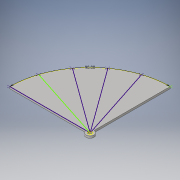
# Autodesk Inventor part: swiweller
Saved by Autodesk Inventor 2016 SP2 (Build 200236200, 236)
## iProperties
Created: 2017-09-03
Part Number: swiweller
Material: Generic
Document SubType Name: Modeling
Designer: Kartikye
Density: 1 g/cm^3
Appearance: Default
Author: Kartikye
Autodesk Inventor part; units mm, degrees
ref_plane "YZ Plane" through (0, 0, 0) normal (1, 0, 0) x (0, 1, 0)
ref_plane "XZ Plane" through (0, 0, 0) normal (0, 1, 0) x (-1, 0, 0)
ref_plane "XY Plane" through (0, 0, 0) normal (0, 0, 1) x (1, 0, 0)
sketch "Sketch5" plane through (0, 0, 0) normal (0, 1, 0) x (-1, 0, 0)
  line L0 (0, 0) -> (127, 0) construction
  circle A0 centre (0, 0) radius 127
  line L1 (0, 0) -> (127, 0)
  line L2 (0, 0) -> (0, -127)
  dimension "d27" = 254
  constraints: 6 end point, 2 horizontal, 1 coincident, 1 vertical, 1 vertical alignment, 2 other
extrude "Extrusion2" add sketch "Sketch5" along normal blind 3.175
sketch "Sketch6" plane through (0, 3.175, 0) normal (0, 1, 0) x (1, 0, 0)
  circle A0 centre (0, 0) radius 127 projected
  line L0 (0, 0) -> (-127, 0)
  line L1 (0, 0) -> (0, 127)
  line L2 (-127, 0) -> (-147.1811, -31.5463)
  line L3 (-147.1811, -31.5463) -> (-90.1509, -154.4564)
  line L4 (-90.1509, -154.4564) -> (47.5084, -160.3561)
  line L5 (47.5084, -160.3561) -> (160.365, -93.0014)
  line L6 (160.365, -93.0014) -> (183.4453, 199.208)
  line L7 (183.4453, 199.208) -> (0, 127)
  constraints: 16 end point, 2 point on circle, 1 horizontal, 1 perpendicular
extrude "Extrusion3" cut sketch "Sketch6" against normal blind 3.175 contours A0 L0 L1 picked at (43.7214, -72.324)
sketch "Sketch9" plane through (0, 3.175, 0) normal (0, 1, 0) x (1, 0, 0)
  circle A0 centre (0, 0) radius 6.35
  circle A1 centre (0, 0) radius 3.175
  dimension "d37" = 12.7
  dimension "d38" = 6.35
  constraints: 2 centre point, 2 coincident
  measures "d37" diameter of A0
  measures "d38" diameter of A1
extrude "Extrusion5" add sketch "Sketch9" against normal blind 3.175
sketch "Sketch10" plane through (0, 3.175, 0) normal (0, 1, 0) x (1, 0, 0)
  circle A0 centre (0, 0) radius 3.175
  dimension "d41" = 6.35
  constraints: 1 centre point, 1 coincident
  measures "d41" diameter of A0
extrude "Extrusion6" cut sketch "Sketch10" against normal blind 6.35
sketch "Sketch11" plane through (0, 3.175, 0) normal (0, 1, 0) x (1, 0, 0)
  arc A0 (0, 127) -> (-127, 0) centre (0, 0) ccw projected
  arc A1 (0, 127) -> (0, 127) centre (0, 0) ccw
  line L0 (-127, 0) -> (0, 0)
  line L1 (-127, 0) -> (0, 0)
  line L2 (-120.7842, 39.2452) -> (0, 0)
  circle A2 centre (0, 0) radius 3.175 projected
  line L3 (-102.7452, 74.6487) -> (0, 0)
  line L4 (0, 0) -> (-74.6487, 102.7452)
  line L5 (-39.2452, 120.7842) -> (0, 0)
  point P0 (0, 127)
  dimension "d52" = 90
  constraints: 12 end point, 2 coincident, 1 collinear, 1 horizontal, 1 vertical alignment, 9 other
equation "\"d42\" = d41"
body "Solid2"
